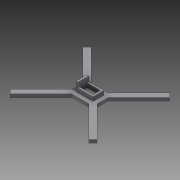
# Autodesk Inventor part: base
Saved by Autodesk Inventor 2020 (Build 240168000, 168)
## iProperties
Created: 2020-02-04
Part Number: base
Material: Generic
Document SubType Name: Modeling
Designer: Wes
Density: 1 g/cm^3
Appearance: Default
Author: Wes
Autodesk Inventor part; units mm, degrees
ref_plane "YZ Plane" through (0, 0, 0) normal (1, 0, 0) x (0, 1, 0)
ref_plane "XZ Plane" through (0, 0, 0) normal (0, 1, 0) x (-1, 0, 0)
ref_plane "XY Plane" through (0, 0, 0) normal (0, 0, 1) x (1, 0, 0)
sketch "Sketch1 - motor_fit" plane through (0, 0, 0) normal (0, 0, 1) x (1, 0, 0)
  line L0 (0, 0) -> (0, 29)
  line L1 (0, 29) -> (18.5, 29)
  line L2 (18.5, 29) -> (18.5, 0)
  line L3 (18.5, 0) -> (0, 0)
  line L4 (9.25, 0) -> (9.25, 3) construction
  line L5 (0, 14.5) -> (3, 14.5) construction
  line L6 (18.5, 14.5) -> (15.5, 14.5) construction
  line L7 (3, 3) -> (15.5, 3)
  line L8 (15.5, 3) -> (15.5, 26)
  line L9 (15.5, 26) -> (3, 26)
  line L10 (3, 26) -> (3, 3)
  dimension "d0" = 29
  dimension "d1" = 18.5
  dimension "d2" = 3
  dimension "d3" = 3
  dimension "d4" = 3
  dimension "d5" = 23
  dimension "d6" = 12.5
  constraints: 22 end point, 6 perpendicular, 3 horizontal, 3 midpoint, 2 vertical
  measures "d0" distance of L0.start L0.end
  measures "d1" distance of L0.end L1.end
  measures "d2" distance of L4.start L4.end
  measures "d3" distance of L5.start L5.end
  measures "d4" distance of L6.start L6.end
  measures "d5" distance of L7.end L8.end
  measures "d6" distance of L8.end L9.end
extrude "Extrusion1" add sketch "Sketch1 - motor_fit" along normal blind 7
sketch "Sketch2 motor_edge" plane through (0, 0, 7) normal (0, 0, 1) x (1, 0, 0)
  line L0 (0, 0) -> (18.5, 0)
  line L1 (18.5, 0) -> (18.5, 3)
  line L2 (18.5, 3) -> (0, 3)
  line L3 (0, 3) -> (0, 0)
  constraints: 8 end point, 2 perpendicular, 1 horizontal
extrude "Extrusion2" add sketch "Sketch2 motor_edge" along normal blind 8.6
sketch "Sketch3 - base_legs" plane through (0, 0, 0) normal (0, 0, -1) x (-1, 0, 0)
  line L0 (-9.25, 29) -> (-9.25, 36) construction
  line L1 (0, 14.5) -> (7, 14.5) construction
  line L2 (-18.5, 13) -> (-25.5, 13) construction
  line L3 (-25.5, 36) -> (7, 36)
  line L4 (-9.25, 0) -> (-9.25, -7) construction
  line L5 (-25.5, -7) -> (-25.5, 36)
  line L6 (-25.5, -7) -> (7, -7)
  line L7 (7, -7) -> (7, 36)
  line L8 (-18.5, 29) -> (-75.0685, 85.5685) construction
  line L9 (-18.5, 36) -> (-71.5684, 89.0684)
  line L10 (-25.5, 29) -> (-78.5684, 82.0684)
  line L11 (-78.5684, 82.0684) -> (-71.5684, 89.0684)
  line L12 (7, 29) -> (60.0684, 82.0684)
  line L13 (0, 36) -> (53.0684, 89.0684)
  line L14 (53.0684, 89.0684) -> (60.0684, 82.0684)
  line L15 (7, 0) -> (60.0684, -53.0684)
  line L16 (0, -7) -> (53.0684, -60.0684)
  line L17 (53.0684, -60.0684) -> (60.0684, -53.0684)
  line L18 (-25.5, 0) -> (-78.5684, -53.0684)
  line L19 (-18.5, -7) -> (-71.5684, -60.0684)
  line L20 (-71.5684, -60.0684) -> (-78.5684, -53.0684)
  dimension "d13" = 7
  dimension "d14" = 7
  dimension "d15" = 7
  dimension "d16" = 32.5
  dimension "d17" = 7
  dimension "d18" = 43
  dimension "d21" = 80
  dimension "d23" = 75.05
  dimension "d24" = 75.05
  dimension "d26" = 75.05
  dimension "d29" = 75.05
  constraints: 42 end point, 8 point on line, 4 horizontal, 3 vertical, 2 perpendicular, 1 parallel
  measures "d13" distance of L0.start L0.end
  measures "d14" distance of L1.start L1.end
  measures "d15" distance of L2.start L2.end
  measures "d16" distance of L3.start L3.end
  measures "d17" distance of L4.start L4.end
  measures "d18" distance of L5.start L3.start
  measures "d21" distance of L8.start L8.end
  measures "d23" distance of L9.start L9.end
  measures "d24" distance of L12.start L12.end
  measures "d26" distance of L15.start L15.end
  measures "d29" distance of L19.start L19.end
extrude "Extrusion3" add sketch "Sketch3 - base_legs" along normal blind 5.5
body "Solid1"
